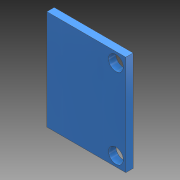
# Autodesk Inventor part: IMU SENSOR
Saved by Autodesk Inventor 2017 (Build 210142000, 142)
## iProperties
Created: 2017-04-01
Part Number: IMU SENSOR
Material: Generic
Document SubType Name: Modeling
Designer: Muchen
Density: 1 g/cm^3
Appearance: Default
Author: Muchen
Autodesk Inventor part; units mm, degrees
ref_plane "YZ Plane" through (0, 0, 0) normal (1, 0, 0) x (0, 1, 0)
ref_plane "XZ Plane" through (0, 0, 0) normal (0, 1, 0) x (-1, 0, 0)
ref_plane "XY Plane" through (0, 0, 0) normal (0, 0, 1) x (1, 0, 0)
sketch "Sketch1" plane through (0, 0, 0) normal (0, 1, 0) x (-1, 0, 0)
  line L0 (0, 0) -> (-16, 0)
  line L1 (-16, 0) -> (-16, -20.26)
  line L2 (-16, -20.26) -> (0, -20.26)
  line L3 (0, -20.26) -> (0, 0)
  circle A0 centre (-14, -18.26) radius 1.5
  circle A1 centre (-14, -2) radius 1.5
  dimension "d0" = 20.26
  dimension "d1" = 16
  dimension "d2" = 3
  dimension "d3" = 2
  dimension "d4" = 2
  dimension "d5" = 2
  constraints: 8 end point, 2 centre point, 2 parallel, 1 equal radius, 1 horizontal, 1 perpendicular, 1 vertical alignment
  measures "d0" distance of L0.end L1.end
  measures "d1" distance of L0.start L0.end
  measures "d2" diameter of A0
  measures "d3" distance from line of L2 A0.centre
  measures "d4" distance from line of L1 A0.centre
  measures "d5" distance from line of L0 A1.centre
extrude "Extrusion1" add sketch "Sketch1" along normal blind 1.5
body "Solid1"
